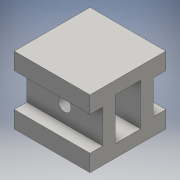
# Autodesk Inventor part: BeamConnectionPoint
Saved by Autodesk Inventor 2016 (Build 200138000, 138)
## iProperties
Created: 2015-11-17
Part Number: BeamConnectionPoint
Material: Generic
Document SubType Name: Modeling
Designer: hesaon
Density: 1 g/cm^3
Appearance: Default
Author: hesaon
Autodesk Inventor part; units mm, degrees
ref_plane "YZ Plane" through (0, 0, 0) normal (1, 0, 0) x (0, 1, 0)
ref_plane "XZ Plane" through (0, 0, 0) normal (0, 1, 0) x (-1, 0, 0)
ref_plane "XY Plane" through (0, 0, 0) normal (0, 0, 1) x (1, 0, 0)
sketch "Sketch1" plane through (0, 0, 0) normal (0, 0, 1) x (1, 0, 0)
  line L0 (0, 0) -> (18, 0)
  line L1 (18, 0) -> (18, 18)
  line L2 (18, 18) -> (0, 18)
  line L3 (0, 18) -> (0, 0)
  dimension "d0" = 18
  dimension "d1" = 18
  constraints: 8 end point, 2 parallel, 1 horizontal, 1 perpendicular
  measures "d0" distance of L2.end L1.end
  measures "d1" distance of L1.end L0.end
extrude "Extrusion1" add sketch "Sketch1" along normal blind 16
sketch "Sketch2" plane through (18, 0, 0) normal (1, 0, 0) x (0, 0, -1)
  line L0 (-16, 0) -> (-12, 0)
  line L1 (0, 0) -> (-16, 0) projected
  line L2 (-12, 0) -> (-12, 3)
  line L3 (-12, 3) -> (-4, 3)
  line L4 (-4, 3) -> (-4, 0)
  line L5 (-16, 0) -> (-16, 18) projected
  line L6 (-16, 18) -> (-12, 18)
  line L7 (0, 18) -> (-16, 18) projected
  line L8 (-12, 15) -> (-4, 15)
  line L9 (-4, 15) -> (-4, 18)
  line L10 (-12, 18) -> (-12, 15)
  dimension "d4" = 4
  dimension "d5" = 3
  dimension "d6" = 8
  dimension "d7" = 4
  dimension "d8" = 8
  dimension "d9" = 3
  constraints: 16 end point, 4 perpendicular, 4 point on line, 1 horizontal, 1 parallel
  measures "d4" distance of L0.start L0.end
  measures "d5" distance of L0.end L2.end
  measures "d6" distance of L2.end L3.end
  measures "d7" distance of L5.end L6.end
  measures "d8" distance of L8.start L8.end
  measures "d9" distance of L6.end L8.start
extrude "Extrusion2" cut sketch "Sketch2" against normal through all
sketch "Sketch3" plane through (18, 0, 0) normal (1, 0, 0) x (0, 0, -1)
  line L0 (-13, 12) -> (-3, 12)
  line L1 (-3, 12) -> (-3, 6)
  line L2 (-3, 6) -> (-13, 6)
  line L3 (-13, 6) -> (-13, 12)
  line L4 (0, 0) -> (0, 18) projected
  line L5 (-16, 0) -> (-16, 18) projected
  line L6 (-4, 15) -> (-12, 15) projected
  line L7 (-12, 3) -> (-4, 3) projected
  dimension "d12" = 3
  dimension "d13" = 3
  dimension "d14" = 3
  dimension "d15" = 3
  constraints: 8 end point, 2 parallel, 1 horizontal, 1 perpendicular
  measures "d12" distance between parallel lines of L4 L1
  measures "d13" distance between parallel lines of L5 L3
  measures "d14" distance between parallel lines of L6 L0
  measures "d15" distance between parallel lines of L2 L7
extrude "Extrusion3" cut sketch "Sketch3" against normal through all
sketch "Sketch4" plane through (18, 15, 12) normal (0, 1, 0) x (1, 0, 0)
  circle A0 centre (-9, 4) radius 1.5
  line L0 (-18, 8) -> (0, 8) projected
  line L1 (-18, 0) -> (-18, 8) projected
  point P0 (-18, 12)
  dimension "d18" = 3
  dimension "d19" = 4
  dimension "d20" = 9
  constraints: 1 centre point
  measures "d18" diameter of A0
  measures "d19" distance from line of A0.centre L0
  measures "d20" distance from line of L1 A0.centre
extrude "Extrusion4" cut sketch "Sketch4" against normal through all
equation "\"d7\" = d4"
equation "\"d8\" = d6"
equation "\"d9\" = d5"
equation "\"d13\" = d12"
equation "\"d15\" = d14"
body "Solid1"
